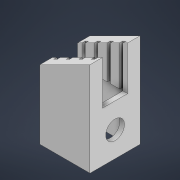
# Autodesk Inventor part: 架
Saved by Autodesk Inventor 2021 (Build 250183000, 183)
## iProperties
Created: 2020-12-09
Part Number: 架
Material: 一般
Document SubType Name: Modeling
Designer: zihon
Density: 1 g/cm^3
Appearance: 預設
Author: zihon
Autodesk Inventor part; units mm, degrees
ref_plane "XZ Plane" through (0, 0, 0) normal (0, 1, 0) x (-1, 0, 0)
ref_plane "XY Plane" through (0, 0, 0) normal (0, 0, 1) x (1, 0, 0)
sketch "草圖1" plane through (0, 0, 0) normal (0, 0, 1) x (1, 0, 0)
  line L0 (0, 0) -> (80, 0)
  line L1 (80, 0) -> (80, 150)
  line L2 (0, 110) -> (0, 0)
  line L3 (80, 150) -> (0, 110)
  line L4 (0, 70) -> (80, 70)
  dimension "d3" = 70
  dimension "d4" = 40
  dimension "d5" = 80
  dimension "d73" = 80
  constraints: 10 end point, 2 perpendicular, 2 point on line, 1 horizontal, 1 parallel
  measures "d3" distance of L0.start L4.start
  measures "d4" distance of L2.start L4.start
  measures "d5" horizontal distance of L1.end L2.start
  measures "d73" distance of L4.end L1.end
extrude "擠出1" add sketch "草圖1" along normal mid plane 80
sketch "草圖5" plane through (0, 0, 40) normal (-1, 0, 0) x (0, 0, 1)
  circle A0 centre (-40, 40) radius 15
  line L0 (-80, 0) -> (0, 0) projected
  line L1 (-40, -30) -> (-40, 180) projected
  point P0 (-40, 0)
  dimension "d24" = 40
  dimension "d25" = 30
  constraints: 1 centre point, 1 point on line
  measures "d24" distance from line of L0 A0.centre
  measures "d25" diameter of A0
extrude "擠出5" cut sketch "草圖5" against normal through all
sketch "草圖11" plane through (0, 0, 0) normal (1, 0, 0) x (0, 1, 0)
  line L0 (150, -40) -> (150, 40) projected
  line L1 (80, -20) -> (150, -20)
  line L2 (150, -20) -> (150, 20)
  line L3 (150, 20) -> (80, 20)
  line L4 (80, 20) -> (80, -20)
  line L5 (80, -20) -> (150, 20) construction
  line L6 (150, -20) -> (80, 20) construction
  line L7 (-28, 0) -> (168, 0) projected
  line L8 (0, -40) -> (0, 40) projected
  point P0 (0, 0)
  point P1 (115, 0)
  point P2 (115, 0)
  dimension "d55" = 40
  dimension "d56" = 80
  constraints: 12 end point, 3 midpoint, 2 parallel, 2 point on line, 1 horizontal, 1 perpendicular
  measures "d55" distance of L2.end L1.end
  measures "d56" distance between parallel lines of L8 L4
extrude "擠出11" cut sketch "草圖11" along normal through all
ref_plane "工作平面5" through (7.5, 0, 0) normal (1, 0, 0) x (0, 1, 0)
sketch "草圖12" plane through (7.5, 0, 0) normal (1, 0, 0) x (0, 1, 0)
  line L0 (0, -40) -> (0, 40) projected
  line L1 (80, -30) -> (0, -30)
  line L2 (0, -30) -> (0, 30)
  line L3 (0, 30) -> (80, 30)
  line L4 (80, 30) -> (80, -30)
  circle A0 centre (40, 0) radius 15 projected
  line L5 (80, -30) -> (0, 30) construction
  line L6 (0, -30) -> (80, 30) construction
  point P0 (0, 0)
  dimension "d60" = 60
  constraints: 12 end point, 2 midpoint, 2 parallel, 1 horizontal, 1 perpendicular, 1 point on line
  measures "d60" distance of L1.end L2.end
extrude "擠出12" cut sketch "草圖12" along normal blind 65
sketch "草圖13" plane through (7.5, 0, 0) normal (1, 0, 0) x (0, 1, 0)
  line L0 (150, -40) -> (150, -20) projected
  line L1 (150, -20) -> (80, -20)
  line L2 (80, -20) -> (80, -25)
  line L3 (80, -25) -> (150, -25)
  line L4 (150, -25) -> (150, -20)
  line L5 (0, 0) -> (140, 0) construction
  line L6 (150, 40) -> (150, 20)
  line L7 (150, 20) -> (80, 20)
  line L8 (80, 25) -> (150, 25)
  line L9 (150, 25) -> (150, 20)
  line L10 (80, 20) -> (80, -20) projected
  line L11 (80, -20) -> (80, 20) projected
  line L12 (80, 20) -> (80, 25)
  dimension "d72" = 5
  constraints: 20 end point, 5 symmetric about line, 2 collinear, 2 horizontal, 2 parallel, 1 perpendicular
  measures "d72" distance between parallel lines of L1 L3
extrude "擠出13" cut sketch "草圖13" along normal blind 5
pattern_linear "矩形陣列3" count 4 spacing 20 along (1, 0, 0) of "擠出13"
